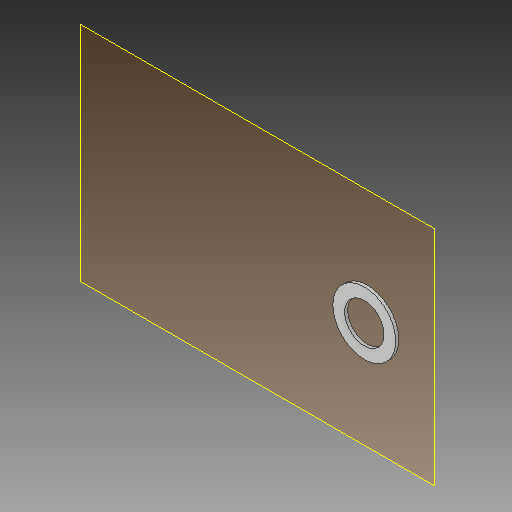
# Autodesk Inventor part: Washer
Saved by Autodesk Inventor 2018 (Build 220112000, 112)
## iProperties
Created: 2016-07-20
Part Number: Washer
Material: Generic
Document SubType Name: Modeling
Designer: User
Density: 1 g/cm^3
Appearance: Default
Mass: 0.0245322 g
Surface Area: 1.24013 cm^2
Volume: 0.0245322 cm^3
Author: User
Autodesk Inventor part; units mm, degrees
ref_plane "YZ Plane" through (0, 0, 0) normal (1, 0, 0) x (0, 1, 0)
ref_plane "XZ Plane" through (0, 0, 0) normal (0, 1, 0) x (-1, 0, 0)
ref_plane "XY Plane" through (0, 0, 0) normal (0, 0, 1) x (1, 0, 0)
ref_plane "Work Plane1" through (0.4707, 0, 0) normal (0, 0, 1) x (1, 0, 0)
sketch "Sketch1" plane through (0.4707, 0, 0) normal (0, 0, 1) x (1, 0, 0)
  circle A0 centre (20.523, 3.1612) radius 2.6 projected
  circle A1 centre (20.523, 3.1612) radius 3.1719
  circle A2 centre (20.523, 3.1612) radius 5.0674
  point P0 (-0.4707, 0)
  constraints: 2 centre point, 2 coincident
extrude "Extrusion1" add sketch "Sketch1" along normal blind 0.5 contours A2
body "Solid1"
